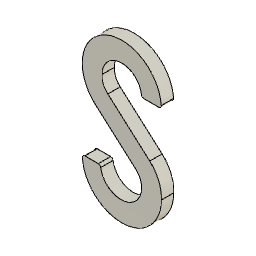
South (Autodesk Fusion 360 design; units mm, degrees)
Autodesk Fusion 360 part; units mm, degrees
note: some values were not read from the file. Set by a fixed rule: which sketch regions a step uses.
sketch "Sketch1" plane through (0, 0, 0) normal (0, 1, 0) x (1, 0, 0)
  line L0 (-19.0076, 0) -> (-12.0684, 0)
  arc A0 (10.16, 0) -> (-10.8108, 1.0933) centre (-0.3734, -0.3734) ccw
  line L1 (0, -40.64) -> (0, -50.8)
  line L2 (19.0076, -40.64) -> (11.3592, -40.64)
  arc A1 (-10.16, -40.64) -> (10.0971, -41.7689) centre (0, -40.64) ccw
  line L3 (-14.3684, -26.2716) -> (7.1842, -7.1842)
  line L4 (-7.1842, -33.4558) -> (14.3684, -14.3684)
  arc A2 (7.1842, -7.1842) -> (10.16, 0) centre (1.2978, -0.5376) ccw
  arc A3 (20.32, 0) -> (-20.2748, 1.3547) centre (0, 0) ccw
  arc A4 (-20.32, -40.64) -> (20.2748, -41.9947) centre (0, -40.64) ccw
  arc A5 (14.3684, -14.3684) -> (20.32, 0) centre (2.5957, -1.0752) ccw
  arc A6 (-7.1842, -33.4558) -> (-10.16, -40.64) centre (-1.2978, -40.1024) ccw
  arc A7 (-14.3684, -26.2716) -> (-20.32, -40.64) centre (0, -40.64) ccw
  arc A8 (20.2748, -41.9947) -> (19.0076, -40.64) centre (19.0076, -41.91) ccw
  arc A9 (11.3592, -40.64) -> (10.0971, -41.7689) centre (11.3592, -41.91) ccw
  arc A10 (-20.2748, 1.3547) -> (-19.0076, 0) centre (-19.0076, 1.27) ccw
  arc A11 (-12.0684, 0) -> (-10.8108, 1.0933) centre (-12.0684, 1.27) ccw
  dimension "d11" = 10.16
  dimension "d15" = 1.27
  constraint coincident L1.end A1
  constraint tangent L3 A2
  constraint tangent L4 A5
  constraint tangent L4 A6
  constraint tangent A4 A7
  constraint tangent L2 A8
  constraint tangent A4 A8
  constraint tangent L2 A9
  constraint tangent A1 A9
  constraint equal A8 A9
  constraint tangent L0 A10
  constraint tangent A3 A10
  constraint equal A8 A10
  constraint tangent L0 A11
  constraint tangent A0 A11
  constraint equal A8 A11
  measures "d11" distance of A3.start A0.start
  measures "d15" radius of A8
extrude "Extrude1" add sketch "Sketch1" along normal blind 6.35
